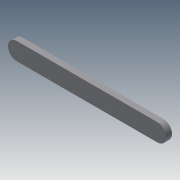
# Autodesk Inventor part: packa_sablona_horni_tahlo
Saved by Autodesk Inventor 2013 (Build 170138000, 138)
## iProperties
Created: 2013-06-15
Part Number: packa_sablona_horni_tahlo
Material: Generic
Document SubType Name: Modeling
Designer: idle-rug
Density: 1 g/cm^3
Author: idle-rug
Autodesk Inventor part; units mm, degrees
ref_plane "YZ Plane" through (0, 0, 0) normal (1, 0, 0) x (0, 1, 0)
ref_plane "XZ Plane" through (0, 0, 0) normal (0, 1, 0) x (-1, 0, 0)
ref_plane "XY Plane" through (0, 0, 0) normal (0, 0, 1) x (1, 0, 0)
sketch "Sketch1" plane through (0, 0, 0) normal (0, 1, 0) x (-1, 0, 0)
  line L0 (-24, -3) -> (24, -3)
  line L1 (24, 3) -> (-24, 3)
  line L2 (-24, -3) -> (24, 3) construction
  line L3 (24, -3) -> (-24, 3) construction
  circle A0 centre (24, 0) radius 0.05
  circle A1 centre (-24, 0) radius 0.05
  arc A2 (24, -3) -> (24, 3) centre (24, 0) ccw
  arc A3 (-24, 3) -> (-24, -3) centre (-24, 0) ccw
  point P0 (0, 0)
  dimension "d0" = 48
  dimension "d1" = 6
  dimension "d3" = 0.1
  dimension "d4" = 0.1
  constraints: 8 end point, 4 centre point, 4 point on circle, 2 midpoint, 1 horizontal, 1 parallel
  measures "d0" distance of L1.end L1.start
  measures "d1" distance of L1.start L0.end
  measures "d3" diameter of A0
  measures "d4" diameter of A1
extrude "Extrusion1" add sketch "Sketch1" along normal blind 2
body "Solid1"
